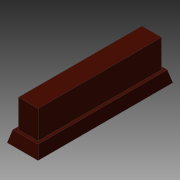
# Autodesk Inventor part: Side2
Saved by Autodesk Inventor 2015 (Build 190159000, 159)
## iProperties
Created: 2016-12-01
Part Number: Side2
Material: Generic
Document SubType Name: Modeling
Designer: Simms
Density: 1 g/cm^3
Appearance: Default
Author: Simms
Autodesk Inventor part; units mm, degrees
ref_plane "YZ Plane" through (0, 0, 0) normal (1, 0, 0) x (0, 1, 0)
ref_plane "XY Plane" through (0, 0, 0) normal (0, 0, 1) x (1, 0, 0)
sketch "Sketch1" plane through (0, 0, 0) normal (0, 1, 0) x (-1, 0, 0)
  line L0 (0, 0) -> (69.85, 0)
  line L1 (69.85, 0) -> (69.85, -304.8)
  line L2 (69.85, -304.8) -> (0, -304.8)
  line L3 (0, -304.8) -> (0, 0)
  dimension "d0" = 69.85
  dimension "d1" = 304.8
  constraints: 8 end point, 2 parallel, 1 horizontal, 1 perpendicular
  measures "d0" distance of L1.end L2.end
  measures "d1" distance of L0.end L1.end
ref_plane "Work Plane1" through (0, 25.4, 0) normal (0, 1, 0) x (-1, 0, 0)
sketch "Sketch2" plane through (0, 25.4, 0) normal (0, 1, 0) x (-1, 0, 0)
  line L0 (0, 0) -> (69.85, 0) projected
  line L1 (69.85, 0) -> (69.85, -304.8) projected
  line L2 (69.85, -304.8) -> (0, -304.8) projected
  line L3 (0, -304.8) -> (0, 0) projected
  line L4 (63.5, -298.45) -> (63.5, -6.35)
  line L5 (63.5, -6.35) -> (6.35, -6.35)
  line L6 (6.35, -6.35) -> (6.35, -298.45)
  line L7 (6.35, -298.45) -> (63.5, -298.45)
  dimension "d3" = 6.35
  constraints: 8 end point, 3 other
  measures "d3" distance between parallel lines of L1 L4
loft "Loft1" add profiles "Sketch1", "Sketch2" contours all / L7 L6 L5 L4
sketch "Sketch3" plane through (-63.5, 25.4, -6.35) normal (0, 1, 0) x (1, 0, 0)
  line L0 (57.15, 0) -> (0, 0) projected
  line L1 (57.15, 292.1) -> (57.15, 0) projected
  line L2 (0, 292.1) -> (57.15, 292.1) projected
  line L3 (0, 0) -> (0, 292.1) projected
  line L4 (50.8, 6.35) -> (6.35, 6.35)
  line L5 (6.35, 285.75) -> (50.8, 285.75)
  line L6 (50.8, 285.75) -> (50.8, 6.35)
  line L7 (6.35, 12.7) -> (44.45, 12.7)
  line L8 (44.45, 12.7) -> (44.45, 279.4)
  line L9 (44.45, 279.4) -> (6.35, 279.4)
  line L10 (6.35, 6.35) -> (6.35, 12.7)
  line L11 (6.35, 279.4) -> (6.35, 285.75)
  circle A0 centre (12.7, 50.8) radius 6.35
  circle A1 centre (12.7, 88.9) radius 6.35
  circle A2 centre (12.7, 127) radius 6.35
  circle A3 centre (12.7, 165.1) radius 6.35
  circle A4 centre (12.7, 203.2) radius 6.35
  circle A5 centre (12.7, 241.3) radius 6.35
  point P0 (63.5, -6.35)
  dimension "d8" = 6.35
  dimension "d9" = 12.7
  dimension "d10" = 12.7
  dimension "d11" = 12.7
  dimension "d12" = 12.7
  dimension "d13" = 6.35
  dimension "d14" = 38.1
  dimension "d17" = 38.1
  constraints: 16 end point, 6 centre point, 1 horizontal, 1 parallel, 1 perpendicular, 1 vertical, 11 other
  measures "d8" distance between parallel lines of L1 L6
  measures "d9" distance between parallel lines of L7 L0
  measures "d10" distance between parallel lines of L2 L9
  measures "d11" distance between parallel lines of L8 L1
  measures "d12" diameter of A0
  measures "d13" distance from line of L10 A0.centre
  measures "d14" distance from line of A0.centre L7
  measures "d17" distance of A0.centre A1.centre
extrude "Extrusion1" add sketch "Sketch3" along normal blind 38.1 contours L4 L10 L7 L8 L9 L11 L5 L6 | A0 | A1 | A2 | A3 | A4 | A5
sketch "Sketch4" plane through (-63.5, 63.5, -6.35) normal (0, 1, 0) x (1, 0, 0)
  line L0 (6.35, 6.35) -> (50.8, 6.35)
  line L1 (50.8, 6.35) -> (50.8, 285.75)
  line L2 (50.8, 285.75) -> (6.35, 285.75)
  line L3 (6.35, 285.75) -> (6.35, 6.35)
  point P0 (63.5, -6.35)
  constraints: 8 end point, 2 parallel, 1 horizontal, 1 perpendicular
extrude "Extrusion2" add sketch "Sketch4" along normal blind 25.4
body "Solid1"
